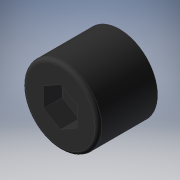
# Autodesk Inventor part: SCHUNK-9965221-Scheibe D4_5
Saved by Autodesk Inventor 2019 (Build 230136000, 136)
## iProperties
Created: 2022-08-29
Part Number: SCHUNK-9965221-Scheibe D4_5
Material: Generic
Catalog Web Link: www.cadenas.de
Description: Scheibe-MPG
Vendor: SCHUNK
Document SubType Name: Modeling
Designer: psAdmin
Manufacturer: SCHUNK
Mass: 0.0517356 g
Surface Area: 0.876784 cm^2
Volume: 0.0517356 cm^3
Density: 1 g/cm^3
Appearance: PSOLRGB-175-175-175
Category: PARTsolutions
Company: SCHUNK
Title: SCHUNK-9965221-Scheibe D4_5
Author: Cadenas PARTsolutions
Comments: MPG
PSOL_IDENT_0: {$CADENAS_DATA/23d-libs/schunk/greifsysteme/greifmodule/greifmodule_pneumatisch/2_finger_parallelgre
PSOL_IDENT_1: ifer/2_finger_kleinteilegreifer/mpg/mpg_scheibe.prj},196 {VTYP=3D},{NB=SCHUNK-9965221-Scheibe D4_5},
PSOL_IDENT_2: {LINA=SCHUNK-9965221-Scheibe D4_5},{NN=Scheibe},{DATE=22.12.2021 07:16:38},{GEOMDATE=14.11.2019 12:1
PSOL_IDENT_3: 1:08},{VERSION=},{LINEID=120},{WBVAR=},{WBNUMERIC=}  {NB=SCHUNK-9965221-Scheibe D4_5},{LINA=SCHUNK-9
PSOL_IDENT_4: 965221-Scheibe D4_5},{KT=DUMMY},{IDNR=9965221},{TYP=Scheibe D4_5},{DZYL=4.500},{HZYL=2.500},{SW=2.00
PSOL_IDENT_5: 0},{TSW=1.100},{DSA=4.500},{HS=1.000},{DSI=2.600},{TYP1=4.000}
NB: SCHUNK-9965221-Scheibe D4_5
NN: Scheibe
NT: MPG
NBSYN: SCHUNK-$IDNR.-$TYP.
LINA: SCHUNK-9965221-Scheibe D4_5
CATALOG: SCHUNK
IDNR: 9965221
TYP: Scheibe D4_5
DZYL: 4.5
HZYL: 2.5
SW: 2
TSW: 1.1
DSA: 4.5
HS: 1
DSI: 2.6
TYP1: 4
SUPPLIER: SCHUNK
ARTICLENO: SCHUNK-9965221-Scheibe D4_5
BOMINFO: SCHUNK-9965221-Scheibe D4_5
CREATOR: CADENAS GmbH
Autodesk Inventor part; units mm, degrees
sketch "Sketch_1" plane through (0, 0, 0) normal (0, 1, 0) x (-1, 0, 0)
  line L0 (0, 3.5) -> (0, 0)
  line L1 (0, 0) -> (-2.25, 0)
  line L2 (-2.25, 0) -> (-2.25, 3.3)
  arc A0 (-2.05, 3.5) -> (-2.25, 3.3) centre (-2.05, 3.3) ccw
  line L3 (-2.05, 3.5) -> (0, 3.5)
  line L4 (0, 3.5) -> (0, 0)
  constraints: 10 end point, 2 point on circle, 1 centre point
revolve "Revolution1" add sketch "Sketch_1" angle 360 about axis through (0, 0, 3.5) along (0, 0, 1)
sketch "Sketch_3" plane through (0, 0, 3.5) normal (0, 0, 1) x (1, 0, 0)
  line L0 (-1, -0.5774) -> (0, -1.1547)
  line L1 (0, -1.1547) -> (1, -0.5774)
  line L2 (1, -0.5774) -> (1, 0.5774)
  line L3 (1, 0.5774) -> (0, 1.1547)
  line L4 (0, 1.1547) -> (-1, 0.5774)
  line L5 (-1, 0.5774) -> (-1, -0.5774)
  constraints: 12 end point
extrude "Extrusion1" cut sketch "Sketch_3" against normal blind 1.1
ref_plane "hal_XY" through (0, 0, 0) normal (0, 0, 1) x (1, 0, 0)
ref_plane "hal_YZ" through (0, 0, 0) normal (1, 0, 0) x (0, 1, 0)
ref_plane "hal_ZX" through (0, 0, 0) normal (0, 1, 0) x (0, 0, 1)
body "Solid1"
